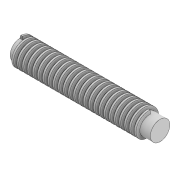
# Autodesk Inventor part: LeadScrew
Saved by Autodesk Inventor 2020 (Build 240168000, 168)
## iProperties
Created: 2023-03-22
Part Number: LeadScrew
Material: Generic
Document SubType Name: Modeling
Designer: ADMIN
Density: 1 g/cm^3
Appearance: Default
Autodesk Inventor part; units mm, degrees
ref_plane "YZ Plane" through (0, 0, 0) normal (1, 0, 0) x (0, 1, 0)
ref_plane "XZ Plane" through (0, 0, 0) normal (0, 1, 0) x (-1, 0, 0)
ref_plane "XY Plane" through (0, 0, 0) normal (0, 0, 1) x (1, 0, 0)
sketch "Sketch1" plane through (0, 0, 0) normal (0, 0, 1) x (1, 0, 0)
  point P0 (0, 0)
sketch "UNNAMED_LEVEL_1" plane through (0, 0, 0) normal (0, 0, 1) x (1, 0, 0)
  line L0 (-2, 7.6435) -> (-1.333, 7.6435)
  line L1 (-1.333, 7.6435) -> (-0.7217, 9.925)
  line L2 (-0.7217, 9.925) -> (0, 9.925)
  line L3 (0, 9.925) -> (0.7217, 9.925)
  line L4 (0.7217, 9.925) -> (1.333, 7.6435)
  line L5 (1.333, 7.6435) -> (2, 7.6435)
  line L6 (1.333, 7.6435) -> (-1.333, 7.6435)
  constraints: 14 end point, 6 horizontal, 14 other
sketch "Sketch3" plane through (0, 0, 0) normal (0, 0, 1) x (1, 0, 0)
  line L0 (-1.333, 7.6435) -> (108.667, 7.6435)
  line L1 (108.667, 7.6435) -> (108.667, -7.6435)
  line L2 (108.667, -7.6435) -> (-1.333, -7.6435)
  line L3 (-1.333, -7.6435) -> (-1.333, 7.6435)
  line L4 (-1.333, 0) -> (108.667, 0)
  point P0 (0, 0)
  dimension "d0" = 110
  constraints: 10 end point, 2 midpoint, 2 parallel, 1 horizontal, 1 horizontal alignment, 1 perpendicular
  measures "d0" distance of L0.start L0.end
revolve "Revolution1" add sketch "Sketch3" angle 360 about axis through (-1.333, 0, 0) along (1, 0, 0) contours L0 L1 L4 L3
sketch "Sketch4" plane through (0, 0, 0) normal (0, 0, 1) x (1, 0, 0)
  line L0 (-1.333, 7.6435) -> (-0.7217, 9.925) projected
  line L1 (-0.7217, 9.925) -> (0, 9.925) projected
  line L2 (0, 9.925) -> (0.7217, 9.925) projected
  line L3 (0.7217, 9.925) -> (1.333, 7.6435) projected
  line L4 (1.333, 7.6435) -> (-1.333, 7.6435) projected
  point P0 (0, 0)
coil "Coil1" sketch "Sketch4" operation add axis through (-10, 0, 0) along (1, 0, 0) pitch 4 turns 25 hand left
body "Solid1"
